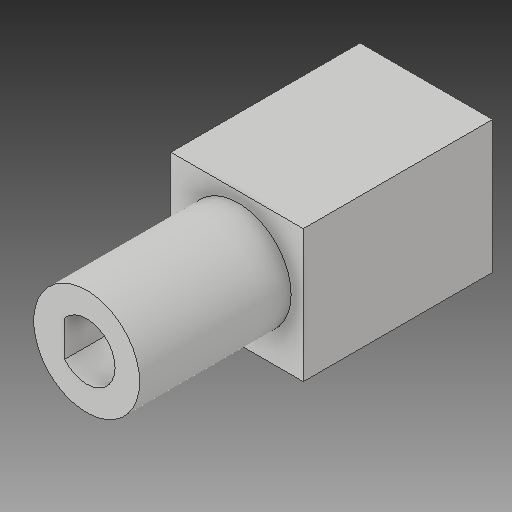
# Autodesk Inventor part: Motor Connection
Saved by Autodesk Inventor 2017 (Build 210142000, 142)
## iProperties
Created: 2017-02-01
Part Number: Motor Connection
Material: Generic
Document SubType Name: Modeling
Designer: aribu
Density: 1 g/cm^3
Appearance: Default
Author: aribu
Autodesk Inventor part; units mm, degrees
ref_plane "YZ Plane" through (0, 0, 0) normal (1, 0, 0) x (0, 1, 0)
ref_plane "XZ Plane" through (0, 0, 0) normal (0, 1, 0) x (-1, 0, 0)
ref_plane "XY Plane" through (0, 0, 0) normal (0, 0, 1) x (1, 0, 0)
sketch "Sketch1" plane through (0, 0, 0) normal (0, 0, 1) x (1, 0, 0)
  line L0 (-4.5134, 4.2398) -> (4.3766, 4.2398)
  line L1 (4.3766, 4.2398) -> (4.3766, -4.6502)
  line L2 (4.3766, -4.6502) -> (-4.5134, -4.6502)
  line L3 (-4.5134, -4.6502) -> (-4.5134, 4.2398)
  point P0 (0, 0)
  dimension "d0" = 8.89
  dimension "d1" = 8.89
  constraints: 8 end point, 2 parallel, 1 horizontal, 1 perpendicular
  measures "d0" distance of L0.start L0.end
  measures "d1" distance of L2.end L0.start
extrude "Extrusion1" add sketch "Sketch1" along normal blind 12.7
sketch "Sketch3" plane through (0, 0, 12.7) normal (0, 0, 1) x (1, 0, 0)
  circle A0 centre (0, 0) radius 3.556
  arc A1 (-1.4785, -1.2013) -> (-1.4785, 1.2013) centre (0, 0) ccw
  line L0 (-1.4785, 1.2013) -> (-1.4785, -1.2013)
  dimension "d12" = 3.81
  dimension "d13" = 7.112
  constraints: 2 centre point, 2 coincident, 2 end point, 2 point on circle, 1 vertical
  measures "d12" diameter of A1
  measures "d13" diameter of A0
extrude "Extrusion3" add sketch "Sketch3" along normal blind 10.16
body "Solid1"
